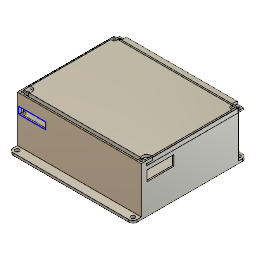
kkClave_Logic_Enclosure (Autodesk Fusion 360 design; units mm, degrees)
Autodesk Fusion 360 part; units mm, degrees
note: some values were not read from the file. Set by a fixed rule: which face or edge a step refers to.
sketch "Case_base" plane through (0, 0, 0) normal (0, 1, 0) x (1, 0, 0)
  line L0 (33, 23) -> (-33, 23)
  line L1 (-33, 23) -> (-33, -23)
  line L2 (-33, -23) -> (33, -23)
  line L3 (33, -23) -> (33, 23)
  line L4 (33, 23) -> (-33, -23) construction
  line L5 (-33, 23) -> (33, -23) construction
  line L6 (-53, 31) -> (41, 31)
  line L7 (41, 31) -> (41, -31)
  line L8 (41, -31) -> (-53, -31)
  line L9 (-53, -31) -> (-53, 31)
  line L10 (-54.7, 32.7) -> (42.7, 32.7)
  line L11 (42.7, 32.7) -> (42.7, -32.7)
  line L12 (42.7, -32.7) -> (-54.7, -32.7)
  line L13 (-54.7, -32.7) -> (-54.7, 32.7)
  line L14 (-54.7, 32.7) -> (42.7, 32.7)
  line L15 (42.7, 32.7) -> (42.7, 37.7)
  line L16 (37.7, 42.7) -> (-49.7, 42.7)
  line L17 (-54.7, 37.7) -> (-54.7, 32.7)
  line L18 (-54.7, -32.7) -> (42.7, -32.7)
  line L19 (42.7, -32.7) -> (42.7, -37.7)
  line L20 (37.7, -42.7) -> (-49.7, -42.7)
  line L21 (-54.7, -37.7) -> (-54.7, -32.7)
  line L22 (-54.7, 37.7) -> (42.7, 37.7)
  line L23 (-54.7, -37.7) -> (42.7, -37.7)
  line L24 (-49.7, 32.7) -> (-49.7, 42.7)
  line L25 (-49.7, -32.7) -> (-49.7, -42.7)
  line L26 (37.7, 32.7) -> (37.7, 42.7)
  line L27 (37.7, -32.7) -> (37.7, -42.7)
  circle A0 centre (-49.7, 37.7) radius 2.5
  circle A1 centre (37.7, 37.7) radius 2.5
  circle A2 centre (-49.7, -37.7) radius 2.5
  circle A3 centre (37.7, -37.7) radius 2.5
  arc A4 (-49.7, 42.7) -> (-54.7, 37.7) centre (-49.7, 37.7) ccw
  arc A5 (42.7, 37.7) -> (37.7, 42.7) centre (37.7, 37.7) ccw
  arc A6 (-54.7, -37.7) -> (-49.7, -42.7) centre (-49.7, -37.7) ccw
  arc A7 (37.7, -42.7) -> (42.7, -37.7) centre (37.7, -37.7) ccw
  circle A8 centre (-33, 23) radius 2.5
  circle A9 centre (33, 23) radius 2.5
  circle A10 centre (-33, -23) radius 2.5
  circle A11 centre (33, -23) radius 2.5
  circle A12 centre (-33, 23) radius 1
  circle A13 centre (33, 23) radius 1
  circle A14 centre (-33, -23) radius 1
  circle A15 centre (33, -23) radius 1
  line L28 (-53, 31) -> (-36.3492, 31) construction
  line L29 (41, 31) -> (69.1579, 31) construction
  line L30 (-53, -31) -> (-39.5464, -31) construction
  line L31 (41, -31) -> (65.2339, -31) construction
  circle A16 centre (-51.55, 29.55) radius 1.45
  circle A17 centre (-51.55, 29.55) radius 2.95
  circle A18 centre (39.55, 29.55) radius 1.45
  circle A19 centre (39.55, 29.55) radius 2.95
  circle A20 centre (-51.55, -29.55) radius 1.45
  circle A21 centre (-51.55, -29.55) radius 2.95
  circle A22 centre (39.55, -29.55) radius 1.45
  circle A23 centre (39.55, -29.55) radius 2.95
  point P0 (-33, 23)
  point P1 (33, 23)
  point P2 (33, -23)
  point P3 (-33, -23)
  point P4 (-49.7, 37.7)
  point P5 (37.7, 37.7)
  point P6 (-49.7, -37.7)
  point P7 (37.7, -37.7)
  point P8 (-53, 31)
  point P9 (41, 31)
  point P10 (-53, -31)
  point P11 (41, -31)
  dimension "d1" = 46
  dimension "d2" = 66
  dimension "d11" = 20
  dimension "d12" = 8
  dimension "d13" = 8
  dimension "d14" = 8
  dimension "d16" = 1.7
  dimension "d17" = 1.7
  dimension "d18" = 1.7
  dimension "d19" = 1.7
  dimension "d21" = 10
  dimension "d22" = 10
  dimension "d23" = 5
  dimension "d24" = 5
  dimension "d25" = 5
  dimension "d26" = 5
  dimension "d27" = 5
  dimension "d28" = 5
  dimension "d30" = 5
  dimension "d31" = 5
  dimension "d32" = 5
  dimension "d33" = 5
  dimension "d34" = 5
  dimension "d35" = 5
  dimension "d36" = 5
  dimension "d37" = 5
  dimension "d41" = 5
  dimension "d42" = 5
  dimension "d43" = 5
  dimension "d44" = 5
  dimension "d45" = 2
  dimension "d46" = 2
  dimension "d47" = 2
  dimension "d48" = 2
  dimension "d57" = 2.9
  dimension "d58" = 5.9
  dimension "d61" = 2.9
  dimension "d62" = 5.9
  dimension "d64" = 2.9
  dimension "d65" = 5.9
  dimension "d67" = 2.9
  dimension "d68" = 5.9
  dimension "d70" = 1.45
  dimension "d71" = 1.45
  dimension "d72" = 1.45
  dimension "d73" = 1.45
  dimension "d74" = 1.45
  dimension "d75" = 1.45
  dimension "d76" = 1.45
  dimension "d77" = 1.45
  constraint perpendicular L0 L1
  constraint parallel L0 L2
  constraint parallel L1 L3
  constraint horizontal L0
  constraint coincident L4 origin
  constraint coincident L5 origin
  constraint horizontal L6
  constraint perpendicular L6 L7
  constraint perpendicular L7 L8
  constraint perpendicular L6 L9
  constraint coincident P0 L0.end
  constraint coincident L0.start L3.end
  constraint coincident P2 L2.end
  constraint coincident L1.end L2.start
  constraint horizontal L10
  constraint perpendicular L10 L11
  constraint perpendicular L11 L12
  constraint perpendicular L10 L13
  constraint perpendicular L14 L15
  constraint parallel L14 L16
  constraint parallel L15 L17
  constraint perpendicular L18 L19
  constraint parallel L18 L20
  constraint parallel L19 L21
  constraint coincident L17 L22.start
  constraint perpendicular L17 L22
  constraint coincident L15 L22.end
  constraint coincident L21 L23.start
  constraint perpendicular L21 L23
  constraint coincident L19 L23.end
  constraint coincident L10 L24.start
  constraint perpendicular L10 L24
  constraint coincident L16 L24.end
  constraint coincident L18 L25.start
  constraint coincident L20 L25.end
  constraint perpendicular L20 L25
  constraint coincident L14 L26.start
  constraint perpendicular L14 L26
  constraint coincident L16 L26.end
  constraint coincident L18 L27.start
  constraint coincident L20 L27.end
  constraint perpendicular L20 L27
  constraint midpoint L24 P4
  constraint midpoint L26 P5
  constraint midpoint L25 P6
  constraint midpoint L27 P7
  constraint coincident P4 A0.centre
  constraint coincident P5 A1.centre
  constraint coincident P6 A2.centre
  constraint coincident P7 A3.centre
  constraint tangent L16 A4
  constraint tangent L17 A4
  constraint tangent L15 A5
  constraint tangent L16 A5
  constraint tangent L20 A6
  constraint tangent L21 A6
  constraint tangent L19 A7
  constraint tangent L20 A7
  constraint coincident P1 L0.start
  constraint coincident P3 L1.end
  constraint coincident P8 L6.start
  constraint coincident P9 L6.end
  constraint coincident L8.end L9.start
  constraint coincident P11 L7.end
  constraint horizontal L28
  constraint horizontal L29
  constraint coincident P10 L8.end
  constraint horizontal L30
  constraint horizontal L31
  constraint concentric A16 A17
  constraint concentric A18 A19
  constraint concentric A20 A21
  constraint concentric A22 A23
  measures "d1" distance of P0 L1.end
  measures "d2" distance of L1.end P2
  measures "d11" distance of L1 L9
  measures "d12" distance of L0 L6
  measures "d13" distance of L3 L7
  measures "d14" distance of L2 L8
  measures "d16" distance of L9 L13
  measures "d17" distance of L6 L10
  measures "d18" distance of L7 L11
  measures "d19" distance of L8 L12
  measures "d21" distance of L14 L16
  measures "d22" distance of L12 L20
  measures "d23" distance of L10 L22
  measures "d24" distance of L12 L23
  measures "d25" distance of L17 L24
  measures "d26" distance of L15 L26
  measures "d27" distance of L21 L25
  measures "d28" distance of L19 L27
  measures "d30" diameter of A0
  measures "d31" diameter of A1
  measures "d32" diameter of A2
  measures "d33" diameter of A3
  measures "d34" radius of A4
  measures "d35" radius of A5
  measures "d36" radius of A6
  measures "d37" radius of A7
  measures "d41" diameter of A8
  measures "d42" diameter of A9
  measures "d43" diameter of A10
  measures "d44" diameter of A11
  measures "d45" diameter of A12
  measures "d46" diameter of A13
  measures "d47" diameter of A14
  measures "d48" diameter of A15
  measures "d57" diameter of A16
  measures "d58" diameter of A17
  measures "d61" diameter of A18
  measures "d62" diameter of A19
  measures "d64" diameter of A20
  measures "d65" diameter of A21
  measures "d67" diameter of A22
  measures "d68" diameter of A23
  measures "d70" distance of L7 A18.centre
  measures "d71" distance of L6 A18.centre
  measures "d72" distance of L6 A16.centre
  measures "d73" distance of L9 A16.centre
  measures "d74" distance of L9 A20.centre
  measures "d75" distance of L8 A20.centre
  measures "d76" distance of L8 A22.centre
  measures "d77" distance of L7 A22.centre
extrude "Extrude1" add sketch "Case_base" against normal blind 3 contours L0 L1 A8 A12 | L0 L1 A8 A12 | L0 L1 L2 L3 A8 A9 A10 A11 | L0 L1 A12 | L0 L1 A12 | L0 L3 A9 A13 | L0 L3 A9 A13 | L0 L3 A13 | L0 L3 A13 | L1 L2 A10 A14 | L1 L2 A10 A14 | L2 L3 A11 A15 | L2 L3 A11 A15 | L1 L2 A14 | L1 L2 A14 | L2 L3 A15 | L2 L3 A15 | L6 L9 A17 | L6 L9 A16 | L6 L9 A16 A17 | A16 | L6 L7 L8 L9 A17 A19 A21 A23 | L6 L7 A19 | L6 L7 A18 A19 | L8 L9 A20 A21 | L8 L9 A21 | L6 L7 A18 | A18 | L8 L9 A20 | A20 | L7 L8 A23 | L7 L8 A22 A23 | A22 | L7 L8 A22 | L10 L14 L17 L22 L24 A0 | L10 L11 L12 L13 L14 L18 | L10 L14 L22 L24 L26 A0 A1 | L12 L18 L21 L23 L25 A2 | L22 L24 A0 A4 | L10 L14 L15 L22 L26 A1 | L12 L18 L23 L25 L27 A2 A3 | L23 L25 A2 A6 | L16 L22 L24 L26 A0 A1 | L12 L18 L19 L23 L27 A3 | L20 L23 L25 L27 A2 A3 | L22 L26 A1 A5 | L23 L27 A3 A7 makes body 1
extrude "Extrude2" cut sketch "Case_base" against normal through all contours L0 L1 A12 | L0 L1 A12 | L0 L3 A13 | L0 L3 A13 | L1 L2 A14 | L1 L2 A14 | L2 L3 A15 | L2 L3 A15 | A16 | A18 | A20 | A22 bodies 1
extrude "Extrude3" add sketch "Case_base" along normal blind 50 contours L6 L9 A17 | L6 L9 A16 | L6 L9 A16 A17 | L6 L7 A19 | L6 L7 A18 A19 | L8 L9 A20 A21 | L8 L9 A21 | L6 L7 A18 | L8 L9 A20 | L7 L8 A23 | L7 L8 A22 A23 | L7 L8 A22 | L10 L11 L12 L13 L14 L18 bodies 1
sketch "Cable_coutouts" plane through (-54.7, 0, 0) normal (-1, 0, 0) x (0, 0, 1)
  line L0 (-32.7, 0) -> (-37.7, 0)
  line L1 (-37.7, 0) -> (-37.7, -3)
  line L2 (-37.7, -3) -> (37.7, -3)
  line L3 (37.7, -3) -> (37.7, 0)
  line L4 (37.7, 0) -> (32.7, 0)
  line L5 (32.7, 0) -> (32.7, 50)
  line L6 (32.7, 50) -> (-32.7, 50)
  line L7 (-32.7, 50) -> (-32.7, 0)
  line L8 (0, 59) -> (0, -14)
  line L9 (-15, 3.5) -> (15, 3.5)
  arc A0 (15, 3.5) -> (15, 6.5) centre (15, 5) ccw
  line L10 (15, 6.5) -> (-15, 6.5)
  arc A1 (-15, 6.5) -> (-15, 3.5) centre (-15, 5) ccw
  line L11 (-15, 5) -> (15, 5) construction
  point P0 (-15, 5)
  point P1 (15, 5)
  point P2 (-42, 12)
  dimension "d83" = 30
  dimension "d84" = 3
  constraint vertical L8
  constraint tangent L9 A0
  constraint tangent A0 L10
  constraint parallel L9 L10
  constraint tangent L10 A1
  constraint tangent L9 A1
  constraint coincident P1 A0.centre
  constraint horizontal L11
  constraint coincident P0 A1.centre
  measures "d83" horizontal distance of P0 P1
  measures "d84" diameter of A0
extrude "Extrude4" cut sketch "Cable_coutouts" against normal blind 5 contours L8 L9 A0 L10 | L8 L9 L10 A1 bodies 1
extrude "Extrude5" add sketch "Case_base" along normal blind 3 contours L0 L1 A8 A12 | L0 L1 A8 A12 | L0 L3 A9 A13 | L0 L3 A9 A13 | L1 L2 A10 A14 | L1 L2 A10 A14 | L2 L3 A11 A15 | L2 L3 A11 A15 bodies 1
chamfer "Chamfer1" distance 0.9 angle 45 4 edges at (-35.3308, 0, 22.096) (-35.3308, 0, -23.904) (30.6692, 0, -23.904) (30.6692, 0, 22.096) on bodies 1
sketch "Lid_base" plane through (0, 50, 0) normal (0, 1, 0) x (-1, 0, 0)
  circle A0 centre (-39.55, -29.55) radius 1.45
  circle A1 centre (51.55, -29.55) radius 1.45
  circle A2 centre (51.55, 29.55) radius 1.45
  circle A3 centre (-39.55, 29.55) radius 1.45
  arc A4 (-36.981, -31) -> (-41, -26.981) centre (-39.55, -29.55) ccw
  line L0 (-41, -26.981) -> (-41, 26.981)
  arc A5 (-41, 26.981) -> (-36.981, 31) centre (-39.55, 29.55) ccw
  line L1 (-36.981, 31) -> (48.981, 31)
  arc A6 (48.981, 31) -> (53, 26.981) centre (51.55, 29.55) ccw
  line L2 (53, 26.981) -> (53, -26.981)
  arc A7 (53, -26.981) -> (48.981, -31) centre (51.55, -29.55) ccw
  line L3 (48.981, -31) -> (-36.981, -31)
  line L4 (54.7, -32.7) -> (54.7, 32.7)
  line L5 (54.7, 32.7) -> (-42.7, 32.7)
  line L6 (-42.7, 32.7) -> (-42.7, -32.7)
  line L7 (-42.7, -32.7) -> (54.7, -32.7)
  arc A8 (52.6, -26.3688) -> (48.3688, -30.6) centre (51.55, -29.55) ccw
  line L8 (48.3688, -30.6) -> (-36.3688, -30.6)
  arc A9 (-36.3688, -30.6) -> (-40.6, -26.3688) centre (-39.55, -29.55) ccw
  line L9 (-40.6, -26.3688) -> (-40.6, 26.3688)
  arc A10 (-40.6, 26.3688) -> (-36.3688, 30.6) centre (-39.55, 29.55) ccw
  line L10 (-36.3688, 30.6) -> (48.3688, 30.6)
  arc A11 (48.3688, 30.6) -> (52.6, 26.3688) centre (51.55, 29.55) ccw
  line L11 (52.6, 26.3688) -> (52.6, -26.3688)
  arc A12 (50.6, -24.285) -> (46.285, -28.6) centre (51.55, -29.55) ccw
  line L12 (46.285, -28.6) -> (-34.285, -28.6)
  arc A13 (-34.285, -28.6) -> (-38.6, -24.285) centre (-39.55, -29.55) ccw
  line L13 (-38.6, -24.285) -> (-38.6, 24.285)
  arc A14 (-38.6, 24.285) -> (-34.285, 28.6) centre (-39.55, 29.55) ccw
  line L14 (-34.285, 28.6) -> (46.285, 28.6)
  arc A15 (46.285, 28.6) -> (50.6, 24.285) centre (51.55, 29.55) ccw
  line L15 (50.6, 24.285) -> (50.6, -24.285)
  dimension "d104" = 0.4
  dimension "d105" = 2.4
extrude "Extrude7" add sketch "Lid_base" along normal blind 5 separate body contours A4 L0 A5 L1 A6 L2 A7 L3 | L4 L5 L6 L7 | A8 L8 A9 L9 A10 L10 A11 L11 | A12 L12 A13 L13 A14 L14 A15 L15 makes body 2
sketch "Lid_screw_counterbore" plane through (0, 55, 0) normal (0, 1, 0) x (-1, 0, 0)
  circle A0 centre (51.55, -29.55) radius 1.45
  circle A1 centre (51.55, 29.55) radius 1.45
  circle A2 centre (-39.55, -29.55) radius 1.45
  circle A3 centre (-39.55, 29.55) radius 1.45
  line L0 (-42.7, -32.7) -> (54.7, -32.7)
  line L1 (54.7, -32.7) -> (54.7, 32.7)
  line L2 (54.7, 32.7) -> (-42.7, 32.7)
  line L3 (-42.7, 32.7) -> (-42.7, -32.7)
hole "Hole1" at (-51.55, 55, 29.55) at (-51.55, 55, -29.55) at (39.55, 55, -29.55) at (39.55, 55, 29.55) direction (0, -1, 0) diameter 5.4 depth 3 tip angle 180 counterbore diameter 10 counterbore depth 3 bodies 2
extrude "Extrude8" add sketch "Lid_base" against normal blind 3 contours A8 L8 A9 L9 A10 L10 A11 L11 bodies 2
ref_plane "WorkPlane1" through (0, 0, 0) normal (1, 0, 0) x (0, 1, 0)
split "Split1" by plane through (0, 0, 0) normal (1, 0, 0) bodies 1 makes body 3 at (10.7037, -3, -7.5139)
move_body "Move1" bodies 3 to x (1, 0, 0) y (0, 1, 0) z (0, 0, 1) at (50, 0, 0)
extrude "Extrude9" add 1 faces at (50, -2, -10.3333) along direction (-1, 0, 0) blind 50 on bodies 3 bodies 3 1
split "Split2" by plane through (0, 0, 0) normal (1, 0, 0) bodies 2 makes body 4 at (12.0048, 55, 8.6715)
move_body "Move2" bodies 4 to x (1, 0, 0) y (0, 1, 0) z (0, 0, 1) at (50, 0, 0)
extrude "Extrude10" add 1 faces at (50, 53.3333, 9.5333) along direction (-1, 0, 0) blind 50 on bodies 4 bodies 4 2
ref_plane "WorkPlane2" through (0, 0, 0) normal (0, 0, 1) x (1, 0, 0)
split "Split3" by plane through (0, 0, 0) normal (0, 0, 1) bodies 3 makes body 5 at (12.6667, 33.3333, 32.7)
move_body "Move3" bodies 5 to x (1, 0, 0) y (0, 1, 0) z (0, 0, 1) at (0, 0, 50)
extrude "Extrude11" add 2 faces at (12.6667, -1, 50) (-54.1333, 35.5, 50) along direction (0, 0, -1) blind 50 on bodies 5 bodies 5 3
split "Split4" by plane through (0, 0, 0) normal (0, 0, 1) bodies 4 makes body 6 at (41.0477, 55, 9.0627)
move_body "Move4" bodies 6 to x (1, 0, 0) y (0, 1, 0) z (0, 0, 1) at (0, 0, 50)
extrude "Extrude12" add 1 faces at (-4.2, 53.3333, 50) along direction (0, 0, -1) blind 50 on bodies 6 bodies 6 4
extrude "Extrude13" add 1 faces at (-53.5667, 3.5, 11.6667) along direction (0, 1, 0) blind 3 on bodies 5 bodies 5
extrude "Extrude14" add 1 faces at (-54.1333, 4.5, 65) along direction (0, 0, 1) blind 5 on bodies 5 bodies 5
extrude "Extrude15" add 1 faces at (-54.1333, 4.5, -15) along direction (0, 0, -1) blind 2 on bodies 5 bodies 5
extrude "Extrude16" add 1 faces at (41.6603, 50, 82.1333) along direction (0, 1, 0) blind 5 on bodies 5 bodies 5
move_body "Move5" bodies 5 to x (1, 0, 0) y (0, 1, 0) z (0, 0, 1) at (-0.3521, 0, 5.9897)
move_face "MoveFace1" to x (1, 0, 0) y (0, 1, 0) z (0, 0, 1) at (-6, 0, 0) 5 faces at (-35.1995, 3, 78.2378) (-35.7013, 2.3, 78.1346) (-35.2849, 0.3, 76.566) (-34.3322, -2, 78.7915) (-34.3322, 2, 78.7915) on bodies 5
move_face "MoveFace2" to x (1, 0, 0) y (0, 1, 0) z (0, 0, 1) at (-4, 0, 0) 5 faces at (-35.2849, 0.3, -19.434) (-32.4643, 3, -15.2242) (-34.1492, -1, -16.4065) (-34.1492, 1, -16.4065) (-30.8645, 1.6, -16.7614) on bodies 5
move_face "MoveFace3" to x (1, 0, 0) y (0, 1, 0) z (0, 0, 1) at (0, 0, 48) 20 faces at (-36.0488, 3, -18.3425) (-35.5145, 3, -17.0103) (-35.5084, 1.6, -18.6988) (-35.1253, 2.3, -18.1468) (-35.0786, 1.6, -15.9704) (-38.3493, -2, -17.0851) (-36.3548, 0.1318, -17.0838) (-36.6154, 0.8448, -16.3341) (-36.3542, 0.1325, -16.9445) (-36.3533, 2.6, -16.9605) (-40.4521, 0.3, -17.0103) (-34.4467, 0.3, -18.0915) (-34.4467, 0.3, -15.9292) (-34.0771, 0.1209, -16.8463) (-34.0808, 0.1254, -17.1574) (80.7151, 0.3, -19.434) (85.1355, 2.3, -17.2593) (84.6386, 3, -17.1345) (81.9497, -1, -16.2945) (81.9497, 1, -16.2945) on bodies 5
move_face "MoveFace4" to x (1, 0, 0) y (0, 1, 0) z (0, 0, 1) at (-45, 0, 0) 5 faces at (80.8005, 3, 78.2378) (80.2987, 2.3, 78.1346) (79.6857, 0.3, 79.9034) (81.6678, -2, 78.7915) (81.6678, 2, 78.7915) on bodies 5
move_face "MoveFace5" to x (1, 0, 0) y (0, 1, 0) z (0, 0, 1) at (-38, 0, 0) 4 faces at (84.6386, 3, 30.8655) (79.6857, 0.3, 30.0759) (85.1355, 1.6, 30.7407) (82.1917, -1, 31.8795) on bodies 5
move_face "MoveFace6" to x (1, 0, 0) y (0, 1, 0) z (0, 0, 1) at (5, 0, 0) 6 faces at (35.8005, 3, 78.2378) (36.6678, 2.6, 78.7915) (36.6788, 0.8, 78.7429) (36.6678, -2, 78.7915) (35.3442, 2.3, 78.0186) (35.7151, 0.3, 81.4133) on bodies 5
move_face "MoveFace7" to x (1, 0, 0) y (0, 1, 0) z (0, 0, 1) at (-7, 0, 0) 6 faces at (46.6386, 3, 30.8655) (45.6467, 2.6, 31.0395) (45.6467, 1.6, 31.0395) (45.6467, -2, 31.0395) (47.1355, 1.6, 30.7407) (46.9204, 0.3, 33.0982) on bodies 5
ref_plane "WorkPlane3" through (-39.3521, 3, 78.9897) normal (0, 1, 0) x (1, 0, 0)
sketch "Sketch5" plane through (-55.0521, 0, 0) normal (-1, 0, 0) x (0, 0, 1)
  line L0 (-26.7103, 55) -> (-26.7103, 0)
  line L1 (-26.7103, 0) -> (-31.7103, 0)
  line L2 (-31.7103, 0) -> (-31.7103, -3)
  line L3 (-31.7103, -3) -> (93.6897, -3)
  line L4 (93.6897, -3) -> (93.6897, 0)
  line L5 (93.6897, 0) -> (88.6897, 0)
  line L6 (88.6897, 0) -> (88.6897, 55)
  line L7 (88.6897, 55) -> (-26.7103, 55)
  line L8 (79, 3) -> (69, 3)
  line L9 (69, 3) -> (69, 16)
  line L10 (69, 16) -> (79, 16)
  line L11 (79, 16) -> (79, 3)
  constraint horizontal L8
  constraint vertical L9
  constraint horizontal L10
  constraint vertical L11
extrude "Extrude17" cut sketch "Sketch5" against normal blind 5 contours L8 L9 L10 L11 bodies 5
sketch "Sketch6" plane through (-55.0521, 0, 0) normal (-1, 0, 0) x (0, 0, 1)
  line L0 (69, 3) -> (69, 16)
  line L1 (69, 16) -> (79, 16)
  line L2 (79, 16) -> (79, 3)
  line L3 (79, 3) -> (69, 3)
  line L4 (-26.7103, 55) -> (-26.7103, 0)
  line L5 (-26.7103, 0) -> (-31.7103, 0)
  line L6 (-31.7103, 0) -> (-31.7103, -3)
  line L7 (-31.7103, -3) -> (93.6897, -3)
  line L8 (93.6897, -3) -> (93.6897, 0)
  line L9 (93.6897, 0) -> (88.6897, 0)
  line L10 (88.6897, 0) -> (88.6897, 55)
  line L11 (88.6897, 55) -> (-26.7103, 55)
  line L12 (50.0791, 3) -> (37.9686, 3)
  line L13 (37.9686, 3) -> (37.9686, 13.4261)
  line L14 (37.9686, 13.4261) -> (50.0791, 13.4261)
  line L15 (50.0791, 13.4261) -> (50.0791, 3)
  line L16 (53, 13) -> (35, 13)
  line L17 (35, 13) -> (35, 25)
  line L18 (35, 25) -> (53, 25)
  line L19 (53, 25) -> (53, 13)
  line L20 (35, 33) -> (67, 33)
  line L21 (67, 33) -> (67, 41)
  line L22 (67, 41) -> (35, 41)
  line L23 (35, 41) -> (35, 33)
  constraint horizontal L12
  constraint vertical L13
  constraint horizontal L14
  constraint vertical L15
  constraint horizontal L16
  constraint vertical L17
  constraint horizontal L18
  constraint vertical L19
  constraint horizontal L20
  constraint vertical L21
  constraint horizontal L22
  constraint vertical L23
extrude "Extrude18" cut sketch "Sketch6" against normal blind 5 contours L12 L13 L15 L16 | L13 L14 L15 L16 L17 L18 L19 | L20 L21 L22 L23 bodies 5
extrude "Extrude19" cut 1 faces at (-55.0521, 13.2841, 46.0423) along direction (1, 0, 0) blind 5 on bodies 5 bodies 5
ref_plane "WorkPlane4" through (-54.2021, 33, 51) normal (0, 1, 0) x (0, 0, 1)
ref_plane "WorkPlane6" through (-53.3521, 27.5, 30.9897) normal (1, 0, 0) x (0, 0, -1)
sketch "Sketch7" plane through (0, 0, 88.6897) normal (0, 0, 1) x (1, 0, 0)
  line L0 (-55.0521, 0) -> (92.3479, 0)
  line L1 (92.3479, 0) -> (92.3479, 55)
  line L2 (92.3479, 55) -> (-55.0521, 55)
  line L3 (-55.0521, 55) -> (-55.0521, 0)
  line L4 (-53.35, 33) -> (-21.35, 33)
  line L5 (-21.35, 33) -> (-21.35, 41)
  line L6 (-21.35, 41) -> (-53.35, 41)
  line L7 (-53.35, 41) -> (-53.35, 33)
  dimension "d135" = 32
  constraint horizontal L4
  constraint vertical L5
  constraint horizontal L6
  constraint vertical L7
  measures "d135" distance of L4.start L4.end
ref_plane "WorkPlane5" through (-53.3521, 27.5, 30.9897) normal (1, 0, 0) x (0, 0, -1)
extrude "Extrude20" cut sketch "Sketch7" against normal blind 10 contours L4 L5 L6 L7 bodies 5
sketch "Sketch8" plane through (92.3479, 0, 0) normal (1, 0, 0) x (0, 0, -1)
  line L0 (-88.6897, 55) -> (-88.6897, 0)
  line L1 (-88.6897, 0) -> (-93.6897, 0)
  line L2 (-93.6897, 0) -> (-93.6897, -3)
  line L3 (-93.6897, -3) -> (31.7103, -3)
  line L4 (31.7103, -3) -> (31.7103, 0)
  line L5 (31.7103, 0) -> (26.7103, 0)
  line L6 (26.7103, 0) -> (26.7103, 55)
  line L7 (26.7103, 55) -> (-88.6897, 55)
  line L8 (-82, 33) -> (-50, 33)
  line L9 (-50, 33) -> (-50, 45)
  line L10 (-50, 45) -> (-82, 45)
  line L11 (-82, 45) -> (-82, 33)
  constraint horizontal L8
  constraint vertical L9
  constraint horizontal L10
  constraint vertical L11
extrude "Extrude21" cut sketch "Sketch8" against normal blind 5 contours L8 L9 L10 L11 bodies 5
sketch "Sketch9" plane through (0, 0, 0) normal (0, 1, 0) x (-1, 0, 0)
  line L0 (53.3521, -20.9913) -> (53.3521, 82.9706)
  arc A0 (49.333, 86.9897) -> (53.3521, 82.9706) centre (51.9021, 85.5397) ccw
  line L1 (49.333, 86.9897) -> (-86.6289, 86.9897)
  arc A1 (-90.6479, 82.9706) -> (-86.6289, 86.9897) centre (-89.1979, 85.5397) ccw
  line L2 (-90.6479, 82.9706) -> (-90.6479, -20.9913)
  arc A2 (-86.6289, -25.0103) -> (-90.6479, -20.9913) centre (-89.1979, -23.5603) ccw
  line L3 (-86.6289, -25.0103) -> (49.333, -25.0103)
  arc A3 (53.3521, -20.9913) -> (49.333, -25.0103) centre (51.9021, -23.5603) ccw
  circle A4 centre (39.3521, 78.9897) radius 3.4
  circle A5 centre (37.3521, 30.9897) radius 3.4
  circle A6 centre (-42.6479, 78.9897) radius 3.4
  circle A7 centre (-37.6479, 30.9897) radius 3.4
  circle A8 centre (-80, -15) radius 2.5
  circle A9 centre (-80, -15) radius 1
  circle A10 centre (-45, -15) radius 1
  circle A11 centre (-45, -15) radius 2.5
  circle A12 centre (-10, -15) radius 1
  circle A13 centre (-10, -15) radius 2.5
  circle A14 centre (25, -15) radius 1
  circle A15 centre (25, -15) radius 2.5
  circle A16 centre (-80, 20) radius 1
  circle A17 centre (-80, 20) radius 2.5
  circle A18 centre (-45, 20) radius 1
  circle A19 centre (-45, 20) radius 2.5
  circle A20 centre (-10, 20) radius 1
  circle A21 centre (-10, 20) radius 2.5
  circle A22 centre (25, 20) radius 1
  circle A23 centre (25, 20) radius 2.5
  circle A24 centre (-27.5025, 20) radius 1
  circle A25 centre (-27.5025, 20) radius 2.5
  circle A26 centre (-27.5025, -20) radius 1
  circle A27 centre (-27.5025, -20) radius 2.5
  dimension "d146" = 35
  dimension "d147" = 35
  dimension "d148" = 1
  dimension "d149" = 2.5
  dimension "d150" = 2
  dimension "d151" = 5
  dimension "d154" = -40
  dimension "d155" = -40
  constraint concentric A8 A9
  constraint concentric A24 A25
  measures "d148" radius of A9
  measures "d149" radius of A8
  measures "d150" diameter of A24
  measures "d151" diameter of A25
extrude "Extrude22" add sketch "Sketch9" along normal blind 4 contours A8 | A11 | A13 | A15 | A17 | A19 | A21 | A23 | A25 | A27 bodies 5
extrude "Extrude23" cut 10 faces at (10.2444, 0, -15.2267) (-25.3185, 0, -15.5517) (-25.3185, 0, 19.4483) (10.2444, 0, 19.6739) (27.2582, 0, 20.4232) (45.3296, 0, -14.4969) (44.7374, 0, 20.4696) (79.7557, 0, 20.4232) (79.7519, 0, -14.7236) (27.2545, 0, -19.7236) along direction (0, -1, 0) blind 5 on bodies 5 bodies 5
equation "d1 = PCB_mounting_holes_H" comment "PCB mounting holes W"
equation "d2 = PCB_mounting_holes_W" comment "PCB mounting holes H"
equation "PCB_mounting_holes_H = 46 mm" comment "PCB_mounting_holes_H"
equation "PCB_mounting_holes_W = 66 mm" comment "PCB_mounting_holes_W"
equation "L_PCB_holes_to_wall_padding = 20 mm" comment "L_PCB_holes_to_wall_padding"
equation "R_PCB_holes_to_wall_padding = 8 mm" comment "R_PCB_holes_to_wall_padding"
equation "T_PCB_holes_to_wall_padding = 8 mm" comment "T_PCB_holes_to_wall_padding"
equation "B_PCB_holes_to_wall_padding = 8 mm" comment "B_PCB_holes_to_wall_padding"
equation "d11 = L_PCB_holes_to_wall_padding"
equation "d12 = T_PCB_holes_to_wall_padding"
equation "d13 = R_PCB_holes_to_wall_padding"
equation "d14 = B_PCB_holes_to_wall_padding"
equation "Wall_thickness = 1.7 mm" comment "Wall_thickness"
equation "d16 = Wall_thickness"
equation "d17 = Wall_thickness"
equation "d18 = Wall_thickness"
equation "d19 = Wall_thickness"
equation "Mounting_flange_stickout = 10 mm" comment "Mounting_flange_stickout"
equation "d21 = Mounting_flange_stickout"
equation "d22 = Mounting_flange_stickout"
equation "d23 = Mounting_flange_stickout / 2"
equation "d24 = Mounting_flange_stickout / 2"
equation "d25 = Mounting_flange_stickout / 2"
equation "d26 = Mounting_flange_stickout / 2"
equation "d27 = Mounting_flange_stickout / 2"
equation "d28 = Mounting_flange_stickout / 2"
equation "Mounting_hole_diameter = 5 mm" comment "Mounting_hole_diameter"
equation "d30 = Mounting_hole_diameter"
equation "d31 = Mounting_hole_diameter"
equation "d32 = Mounting_hole_diameter"
equation "d33 = Mounting_hole_diameter"
equation "d34 = Mounting_flange_stickout / 2"
equation "d35 = Mounting_flange_stickout / 2"
equation "d36 = Mounting_flange_stickout / 2"
equation "d37 = Mounting_flange_stickout / 2"
equation "PCB_mounting_post_diameter = 5 mm" comment "PCB_mounting_post_diameter"
equation "PCB_mounting_post_height = 3 mm" comment "PCB_mounting_post_height"
equation "PCB_mounting_post_hole_diameter = 2 mm" comment "PCB_mounting_post_hole_diameter"
equation "d41 = PCB_mounting_post_diameter"
equation "d42 = PCB_mounting_post_diameter"
equation "d43 = PCB_mounting_post_diameter"
equation "d44 = PCB_mounting_post_diameter"
equation "d45 = PCB_mounting_post_hole_diameter"
equation "d46 = PCB_mounting_post_hole_diameter"
equation "d47 = PCB_mounting_post_hole_diameter"
equation "d48 = PCB_mounting_post_hole_diameter"
equation "Case_base_thickness = 3 mm" comment "Case_base_thickness"
equation "d50 = -Case_base_thickness"
equation "Lid_screw_diameter = 2.9 mm" comment "Lid_screw_diameter"
equation "d57 = Lid_screw_diameter"
equation "d58 = Lid_screw_diameter + Lid_screw_diameter_wall_thickness"
equation "Lid_screw_diameter_wall_thickness = 3 mm" comment "Lid_screw_diameter_wall_thickness"
equation "d61 = Lid_screw_diameter"
equation "d62 = Lid_screw_diameter + Lid_screw_diameter_wall_thickness"
equation "d64 = Lid_screw_diameter"
equation "d65 = Lid_screw_diameter + Lid_screw_diameter_wall_thickness"
equation "d67 = Lid_screw_diameter"
equation "d68 = Lid_screw_diameter + Lid_screw_diameter_wall_thickness"
equation "d70 = Lid_screw_diameter - ( Lid_screw_diameter / 2 )"
equation "d71 = Lid_screw_diameter - ( Lid_screw_diameter / 2 )"
equation "d72 = Lid_screw_diameter - ( Lid_screw_diameter / 2 )"
equation "d73 = Lid_screw_diameter - ( Lid_screw_diameter / 2 )"
equation "d74 = Lid_screw_diameter - ( Lid_screw_diameter / 2 )"
equation "d75 = Lid_screw_diameter - ( Lid_screw_diameter / 2 )"
equation "d76 = Lid_screw_diameter - ( Lid_screw_diameter / 2 )"
equation "d77 = Lid_screw_diameter - ( Lid_screw_diameter / 2 )"
equation "Case_height = 50 mm" comment "Case_height"
equation "d80 = Case_height"
equation "d87 = PCB_mounting_post_height"
equation "d89 = PCB_mounting_post_height * 0.3"
equation "Lid_thickness = 5 mm" comment "Lid_thickness"
equation "d93 = Lid_thickness"
equation "Lid_screw_hole_counterbore_depth = 3 mm" comment "Lid_screw_hole_counterbore_depth"
equation "Lid_screw_head_diameter = 10 mm" comment "Lid_screw_head_diameter"
equation "d97 = Lid_screw_hole_counterbore_depth"
equation "d99 = Lid_screw_counterbore_angle"
equation "d100 = Lid_screw_hole_counterbore_depth"
equation "d101 = Lid_screw_head_diameter"
equation "Lid_screw_counterbore_angle = 180 deg" comment "The screw's under-head angle - 180 for flat head, less for angled heads like self tappers"
equation "d106 = -Lid_strengthening_rib_depth"
equation "Lid_strengthening_rib_depth = 3 mm" comment "Lid_strengthening_rib_depth"
named bodies: "Base", "Lid", "Base (1)", "Lid (1)", "Base (1) (1)", "Lid (1) (1)"
